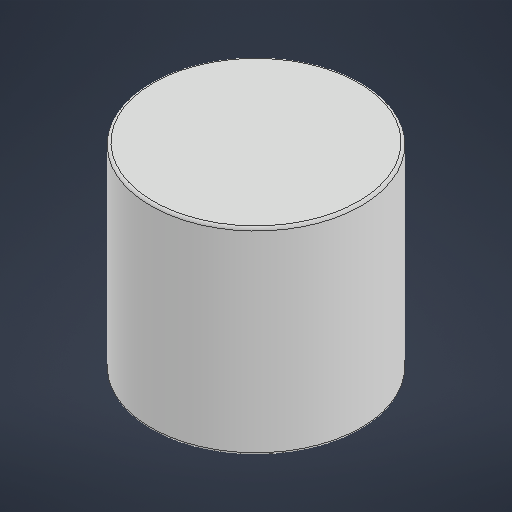
# Autodesk Inventor part: ROLLER_CR_BEARING,REV-ENG
Saved by Autodesk Inventor 2026.2 (Build 302298010, 298A)
## iProperties
Created: 2026-03-05
Part Number: ROLLER_CR_BEARING,REV-ENG
Material: Steel, O1, HT 58-60 Rc
Document SubType Name: Modeling
Designer: 4aida
Density: 7.86 g/cm^3
Appearance: Grey (Light)
Author: 4aida
Autodesk Inventor part; units mm, degrees
ref_plane "YZ Plane" through (0, 0, 0) normal (1, 0, 0) x (0, 1, 0)
ref_plane "XZ Plane" through (0, 0, 0) normal (0, 1, 0) x (-1, 0, 0)
ref_plane "XY Plane" through (0, 0, 0) normal (0, 0, 1) x (1, 0, 0)
sketch "Sketch1" plane through (0, 0, 0) normal (0, 1, 0) x (-1, 0, 0)
  circle A0 centre (0, 0) radius 2
  dimension "d0" = 4
  constraints: 1 centre point, 1 coincident
  measures "d0" diameter of A0
extrude "Extrusion1" add sketch "Sketch1" along normal mid plane 3.75
fillet "Fillet1" radius 0.05 2 edges at (2, 1.875, 0) (2, -1.875, 0)
body "Solid1"
